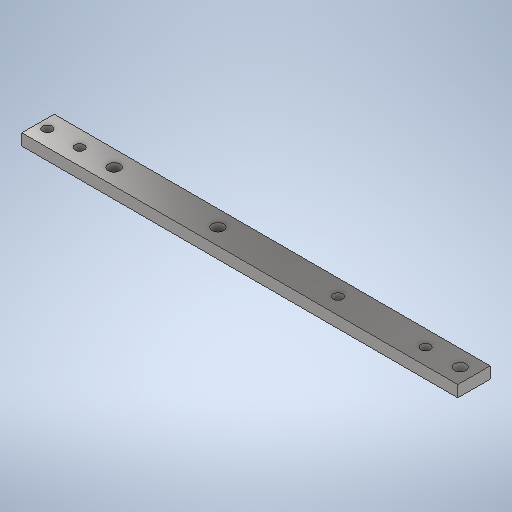
# Autodesk Inventor part: 144
Saved by Autodesk Inventor 2025.1 (Build 291241000, 241)
## iProperties
Created: 2024-08-01
Part Number: 144
Material: Stainless Steel
Document SubType Name: Modeling
Designer: ffogue
Density: 8 g/cm^3
Appearance: Semi-Polished
Author: ffogue
Autodesk Inventor part; units mm, degrees
ref_plane "YZ Plane" through (0, 0, 0) normal (1, 0, 0) x (0, 1, 0)
ref_plane "XZ Plane" through (0, 0, 0) normal (0, 1, 0) x (-1, 0, 0)
ref_plane "XY Plane" through (0, 0, 0) normal (0, 0, 1) x (1, 0, 0)
sketch "Sketch1" plane through (0, 0, 0) normal (0, 0, 1) x (1, 0, 0)
  line L0 (-94.5, 0) -> (94.5, 0)
  line L1 (94.5, 0) -> (94.5, 14)
  line L2 (94.5, 14) -> (-94.5, 14)
  line L3 (-94.5, 14) -> (-94.5, 0)
  point P0 (0, 0)
  point P1 (0, 0)
  dimension "d0" = 14
  dimension "d1" = 189
  constraints: 8 end point, 2 parallel, 1 coincident, 1 horizontal, 1 horizontal alignment, 1 midpoint, 1 perpendicular
  measures "d0" distance between parallel lines of L0 L2
  measures "d1" distance of L1.end L2.end
extrude "Extrusion1" add sketch "Sketch1" along normal blind 5
sketch "Sketch2" plane through (0, 0, 5) normal (0, 0, 1) x (1, 0, 0)
  line L0 (94.5, 0) -> (94.5, 14) projected
  line L1 (-94.5, 0) -> (94.5, 0) projected
  point P0 (0, 0)
  point P1 (-61.5, 7)
  point P2 (-16.5, 7)
  point P3 (88.5, 7)
  dimension "d4" = 6
  dimension "d5" = 7
  dimension "d6" = 105
  dimension "d7" = 45
  constraints: 2 horizontal alignment
  measures "d4" distance from line of L0 point (88.5, 7)
  measures "d5" distance from line of L1 point (88.5, 7)
  measures "d6" distance of point (-16.5, 7) point (88.5, 7)
  measures "d7" distance of point (-16.5, 7) point (-61.5, 7)
hole "Hole1" at (-61.5, 7, 5) at (-16.5, 7, 5) at (88.5, 7, 5) direction (0, 0, -1) diameter 5 depth 5
sketch "Sketch3" plane through (0, 0, 5) normal (0, 0, 1) x (1, 0, 0)
  line L0 (-94.5, 0) -> (94.5, 0) projected
  circle A0 centre (88.5, 7) radius 2.5 projected
  circle A1 centre (-61.5, 7) radius 2.5 projected
  point P0 (0, 0)
  point P1 (73.5, 7)
  point P2 (35.5, 7)
  point P3 (-76.5, 7)
  point P4 (-90.5, 7)
  dimension "d22" = 7
  dimension "d23" = 15
  dimension "d24" = 38
  dimension "d25" = 15
  dimension "d26" = 14
  constraints: 3 horizontal alignment
  measures "d22" distance from line of L0 point (-90.5, 7)
  measures "d23" distance of A0.centre point (73.5, 7)
  measures "d24" distance of point (73.5, 7) point (35.5, 7)
  measures "d25" distance of A1.centre point (-76.5, 7)
  measures "d26" distance of point (-76.5, 7) point (-90.5, 7)
hole "Hole2" at (73.5, 7, 5) at (35.5, 7, 5) at (-76.5, 7, 5) at (-90.5, 7, 5) direction (0, 0, -1) diameter 4 depth 5
body "Solid1"
